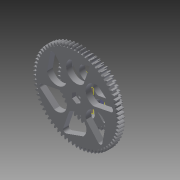
# Autodesk Inventor part: quarterinch-cap
Saved by Autodesk Inventor 2014 (Build 180170000, 170)
## iProperties
Created: 2013-11-06
Part Number: quarterinch-cap
Material: Generic
Document SubType Name: Modeling
Designer: stephen
Density: 1 g/cm^3
Appearance: Default
Author: stephen
Autodesk Inventor part; units mm, degrees
(part 1 of 2)
ref_plane "YZ Plane" through (0, 0, 0) normal (1, 0, 0) x (0, 1, 0)
ref_plane "XZ Plane" through (0, 0, 0) normal (0, 1, 0) x (-1, 0, 0)
ref_plane "XY Plane" through (0, 0, 0) normal (0, 0, 1) x (1, 0, 0)
ref_plane "Work Plane10" through (2.7665, 46.0619, 25.38) normal (0, 0, 1) x (1, 0, 0)
sketch "Sketch15" plane through (2.7665, 46.0619, 25.38) normal (0, 0, 1) x (1, 0, 0)
  line L0 (-0.1767, 42.3028) -> (0.1689, 42.3028)
  arc A0 (0.9579, 39.3583) -> (0.1689, 42.3028) centre (-2.8295, 39.9215) ccw
  line L1 (0.1689, 42.3028) -> (0.9579, 39.3583) construction
  arc A1 (-0.1767, 42.3028) -> (-0.9656, 39.3582) centre (2.8217, 39.9215) ccw
  line L2 (-3.968, 42.1167) -> (-3.6238, 42.1476)
  arc A2 (-2.5741, 39.2858) -> (-3.6238, 42.1476) centre (-6.3966, 39.5071) ccw
  line L3 (-3.6238, 42.1476) -> (-2.5741, 39.2858) construction
  arc A3 (-3.968, 42.1167) -> (-4.4898, 39.1132) centre (-0.7682, 40.0137) ccw
  line L4 (-7.7273, 41.5914) -> (-7.3873, 41.6531)
  arc A4 (-6.0852, 38.8969) -> (-7.3873, 41.6531) centre (-9.9122, 38.7747) ccw
  line L5 (-7.3873, 41.6531) -> (-6.0852, 38.8969) construction
  arc A5 (-7.7273, 41.5914) -> (-7.9778, 38.5532) centre (-4.3519, 39.7837) ccw
  line L6 (-11.4244, 40.7313) -> (-11.0913, 40.8233)
  arc A6 (-9.5474, 38.1948) -> (-11.0913, 40.8233) centre (-13.3481, 37.7301) ccw
  line L7 (-11.0913, 40.8233) -> (-9.5474, 38.1948) construction
  arc A7 (-11.4244, 40.7313) -> (-11.4015, 37.6829) centre (-7.9006, 39.2335) ccw
  line L8 (-15.0295, 39.5433) -> (-14.706, 39.6647)
  arc A8 (-12.9328, 37.1852) -> (-14.706, 39.6647) centre (-16.6764, 36.3817) ccw
  line L9 (-14.706, 39.6647) -> (-12.9328, 37.1852) construction
  arc A9 (-15.0295, 39.5433) -> (-14.7335, 36.5092) centre (-11.3856, 38.3673) ccw
  line L10 (-18.5137, 38.0368) -> (-18.2023, 38.1868)
  arc A10 (-16.2139, 35.8762) -> (-18.2023, 38.1868) centre (-19.8705, 34.7403) ccw
  line L11 (-18.2023, 38.1868) -> (-16.2139, 35.8762) construction
  arc A11 (-18.5137, 38.0368) -> (-17.9468, 35.0415) centre (-14.779, 37.1923) ccw
  line L12 (-21.8487, 36.2242) -> (-21.5521, 36.4014)
  arc A12 (-19.3646, 34.2784) -> (-21.5521, 36.4014) centre (-22.9046, 32.8193) ccw
  line L13 (-21.5521, 36.4014) -> (-19.3646, 34.2784) construction
  arc A13 (-21.8487, 36.2242) -> (-21.0157, 33.2917) centre (-18.0534, 35.7178) ccw
  line L14 (-25.0079, 34.1198) -> (-24.7283, 34.323)
  arc A14 (-22.3593, 32.4046) -> (-24.7283, 34.323) centre (-25.7543, 30.634) ccw
  line L15 (-24.7283, 34.323) -> (-22.3593, 32.4046) construction
  arc A15 (-25.0079, 34.1198) -> (-23.9153, 31.2738) centre (-21.1825, 33.9557) ccw
  line L16 (-27.9657, 31.7408) -> (-27.7055, 31.9681)
  arc A16 (-25.174, 30.2699) -> (-27.7055, 31.9681) centre (-28.3967, 28.2021) ccw
  line L17 (-27.7055, 31.9681) -> (-25.174, 30.2699) construction
  arc A17 (-27.9657, 31.7408) -> (-26.6224, 29.0042) centre (-24.1409, 31.9202) ccw
  line L18 (-30.6983, 29.1062) -> (-30.4595, 29.356)
  arc A18 (-27.7861, 27.8914) -> (-30.4595, 29.356) centre (-30.8104, 25.5431) ccw
  line L19 (-30.4595, 29.356) -> (-27.7861, 27.8914) construction
  arc A19 (-30.6983, 29.1062) -> (-29.1152, 26.501) centre (-26.9051, 29.6277) ccw
  line L20 (-33.1838, 26.2372) -> (-32.9683, 26.5074)
  arc A20 (-30.1744, 25.2884) -> (-32.9683, 26.5074) centre (-32.976, 22.6785) ccw
  line L21 (-32.9683, 26.5074) -> (-30.1744, 25.2884) construction
  arc A21 (-33.1838, 26.2372) -> (-31.3735, 23.7845) centre (-29.4526, 27.0967) ccw
  line L22 (-35.4021, 23.157) -> (-35.2117, 23.4454)
  arc A22 (-32.3197, 22.4818) -> (-35.2117, 23.4454) centre (-34.8761, 19.6312) ccw
  line L23 (-35.2117, 23.4454) -> (-32.3197, 22.4818) construction
  arc A23 (-35.4021, 23.157) -> (-33.3792, 20.8764) centre (-31.7629, 24.3475) ccw
  line L24 (-37.3354, 19.8904) -> (-37.1716, 20.1947)
  arc A24 (-34.2049, 19.4942) -> (-37.1716, 20.1947) centre (-36.4955, 16.4259) ccw
  line L25 (-37.1716, 20.1947) -> (-34.2049, 19.4942) construction
  arc A25 (-37.3354, 19.8904) -> (-35.1162, 17.8003) centre (-33.8176, 21.4023) ccw
  line L26 (-38.968, 16.4636) -> (-38.8322, 16.7814)
  arc A26 (-35.8146, 16.3496) -> (-38.8322, 16.7814) centre (-37.8209, 13.0884) ccw
  line L27 (-38.8322, 16.7814) -> (-35.8146, 16.3496) construction
  arc A27 (-38.968, 16.4636) -> (-36.5704, 14.5808) centre (-35.5999, 18.2847) ccw
  line L28 (-40.2869, 12.9043) -> (-40.1802, 13.2329)
  arc A28 (-37.136, 13.0734) -> (-40.1802, 13.2329) centre (-38.8419, 9.6454) ccw
  line L29 (-40.1802, 13.2329) -> (-37.136, 13.0734) construction
  arc A29 (-40.2869, 12.9043) -> (-37.7302, 11.244) centre (-37.0956, 15.02) ccw
  line L30 (-41.2815, 9.241) -> (-41.2046, 9.5779)
  arc A30 (-38.1584, 9.6919) -> (-41.2046, 9.5779) centre (-39.5502, 6.1248) ccw
  line L31 (-41.2046, 9.5779) -> (-38.1584, 9.6919) construction
  arc A31 (-41.2815, 9.241) -> (-38.5862, 7.8166) centre (-38.2927, 11.6343) ccw
  line L32 (-41.9437, 5.5034) -> (-41.8973, 5.8458)
  arc A32 (-38.8736, 6.2324) -> (-41.8973, 5.8458) centre (-39.94, 2.5549) ccw
  line L33 (-41.8973, 5.8458) -> (-38.8736, 6.2324) construction
  arc A33 (-41.9437, 5.5034) -> (-39.1316, 4.3263) centre (-39.1814, 8.1549) ccw
  line L34 (-42.2681, 1.7214) -> (-42.2526, 2.0666)
  arc A34 (-39.2757, 2.7227) -> (-42.2526, 2.0666) centre (-40.0082, -1.0355) ccw
  line L35 (-42.2526, 2.0666) -> (-39.2757, 2.7227) construction
  arc A35 (-42.2681, 1.7214) -> (-39.3618, 0.8012) centre (-39.7547, 4.6099) ccw
  line L36 (-42.2523, -2.0744) -> (-42.2678, -1.7292)
  arc A36 (-39.3617, -0.8089) -> (-42.2678, -1.7292) centre (-39.7543, -4.6177) ccw
  line L37 (-42.2678, -1.7292) -> (-39.3617, -0.8089) construction
  arc A37 (-42.2523, -2.0744) -> (-39.2752, -2.7304) centre (-40.0079, 1.0278) ccw
  line L38 (-41.8962, -5.8535) -> (-41.9426, -5.5111)
  arc A38 (-39.1307, -4.334) -> (-41.9426, -5.5111) centre (-39.1804, -8.1626) ccw
  line L39 (-41.9426, -5.5111) -> (-39.1307, -4.334) construction
  arc A39 (-41.8962, -5.8535) -> (-38.8723, -6.24) centre (-39.9389, -2.5626) ccw
  line L40 (-41.2029, -9.5855) -> (-41.2798, -9.2486)
  arc A40 (-38.5847, -7.8242) -> (-41.2798, -9.2486) centre (-38.2909, -11.6419) ccw
  line L41 (-41.2798, -9.2486) -> (-38.5847, -7.8242) construction
  arc A41 (-41.2029, -9.5855) -> (-38.1565, -9.6994) centre (-39.5484, -6.1324) ccw
  line L42 (-40.1777, -13.2403) -> (-40.2845, -12.9117)
  arc A42 (-37.728, -11.2514) -> (-40.2845, -12.9117) centre (-37.0932, -15.0274) ccw
  line L43 (-40.2845, -12.9117) -> (-37.728, -11.2514) construction
  arc A43 (-40.1777, -13.2403) -> (-37.1334, -13.0807) centre (-38.8395, -9.6528) ccw
  line L44 (-38.8292, -16.7885) -> (-38.965, -16.4708)
  arc A44 (-36.5676, -14.588) -> (-38.965, -16.4708) centre (-35.5968, -18.2919) ccw
  line L45 (-38.965, -16.4708) -> (-36.5676, -14.588) construction
  arc A45 (-38.8292, -16.7885) -> (-35.8114, -16.3566) centre (-37.8179, -13.0955) ccw
  line L46 (-37.1679, -20.2015) -> (-37.3317, -19.8972)
  arc A46 (-35.1127, -17.8072) -> (-37.3317, -19.8972) centre (-33.8139, -21.4091) ccw
  line L47 (-37.3317, -19.8972) -> (-35.1127, -17.8072) construction
  arc A47 (-37.1679, -20.2015) -> (-34.201, -19.5009) centre (-36.4918, -16.4328) ccw
  line L48 (-35.2074, -23.4519) -> (-35.3978, -23.1635)
  arc A48 (-33.3751, -20.883) -> (-35.3978, -23.1635) centre (-31.7586, -24.354) ccw
  line L49 (-35.3978, -23.1635) -> (-33.3751, -20.883) construction
  arc A49 (-35.2074, -23.4519) -> (-32.3153, -22.4882) centre (-34.8718, -19.6377) ccw
  line L50 (-32.9635, -26.5135) -> (-33.179, -26.2433)
  arc A50 (-31.3688, -23.7906) -> (-33.179, -26.2433) centre (-29.4477, -27.1028) ccw
  line L51 (-33.179, -26.2433) -> (-31.3688, -23.7906) construction
  arc A51 (-32.9635, -26.5135) -> (-30.1694, -25.2944) centre (-32.9711, -22.6845) ccw
  line L52 (-30.4541, -29.3616) -> (-30.693, -29.1118)
  arc A52 (-29.1099, -26.5067) -> (-30.693, -29.1118) centre (-26.8997, -29.6333) ccw
  line L53 (-30.693, -29.1118) -> (-29.1099, -26.5067) construction
  arc A53 (-30.4541, -29.3616) -> (-27.7806, -27.8969) centre (-30.805, -25.5487) ccw
  line L54 (-27.6996, -31.9733) -> (-27.9598, -31.7459)
  arc A54 (-26.6167, -29.0094) -> (-27.9598, -31.7459) centre (-24.1351, -31.9253) ccw
  line L55 (-27.9598, -31.7459) -> (-26.6167, -29.0094) construction
  arc A55 (-27.6996, -31.9733) -> (-25.1681, -30.2748) centre (-28.3908, -28.2072) ccw
  line L56 (-24.722, -34.3275) -> (-25.0016, -34.1244)
  arc A56 (-23.9092, -31.2786) -> (-25.0016, -34.1244) centre (-21.1762, -33.9603) ccw
  line L57 (-25.0016, -34.1244) -> (-23.9092, -31.2786) construction
  arc A57 (-24.722, -34.3275) -> (-22.3529, -32.409) centre (-25.748, -30.6386) ccw
  line L58 (-21.5454, -36.4054) -> (-21.8421, -36.2282)
  arc A58 (-21.0091, -33.2958) -> (-21.8421, -36.2282) centre (-18.0467, -35.7218) ccw
  line L59 (-21.8421, -36.2282) -> (-21.0091, -33.2958) construction
  arc A59 (-21.5454, -36.4054) -> (-19.3578, -34.2822) centre (-22.898, -32.8233) ccw
  line L60 (-18.1953, -38.1902) -> (-18.5067, -38.0402)
  arc A60 (-17.9399, -35.045) -> (-18.5067, -38.0402) centre (-14.772, -37.1956) ccw
  line L61 (-18.5067, -38.0402) -> (-17.9399, -35.045) construction
  arc A61 (-18.1953, -38.1902) -> (-16.2069, -35.8794) centre (-19.8635, -34.7437) ccw
  line L62 (-14.6987, -39.6674) -> (-15.0223, -39.546)
  arc A62 (-14.7263, -36.5121) -> (-15.0223, -39.546) centre (-11.3784, -38.3701) ccw
  line L63 (-15.0223, -39.546) -> (-14.7263, -36.5121) construction
  arc A63 (-14.6987, -39.6674) -> (-12.9254, -37.1878) centre (-16.6692, -36.3844) ccw
  line L64 (-11.0838, -40.8253) -> (-11.4169, -40.7334)
  arc A64 (-11.3941, -37.6852) -> (-11.4169, -40.7334) centre (-7.8931, -39.2355) ccw
  line L65 (-11.4169, -40.7334) -> (-11.3941, -37.6852) construction
  arc A65 (-11.0838, -40.8253) -> (-9.5399, -38.1967) centre (-13.3406, -37.7321) ccw
  line L66 (-7.3796, -41.6545) -> (-7.7196, -41.5928)
  arc A66 (-7.9702, -38.5548) -> (-7.7196, -41.5928) centre (-4.3443, -39.7851) ccw
  line L67 (-7.7196, -41.5928) -> (-7.9702, -38.5548) construction
  arc A67 (-7.3796, -41.6545) -> (-6.0776, -38.8981) centre (-9.9046, -38.7761) ccw
  line L68 (-3.616, -42.1483) -> (-3.9602, -42.1174)
  arc A68 (-4.4821, -39.114) -> (-3.9602, -42.1174) centre (-0.7605, -40.0144) ccw
  line L69 (-3.9602, -42.1174) -> (-4.4821, -39.114) construction
  arc A69 (-3.616, -42.1483) -> (-2.5663, -39.2863) centre (-6.3889, -39.5078) ccw
  line L70 (0.1767, -42.3028) -> (-0.1689, -42.3028)
  arc A70 (-0.9579, -39.3583) -> (-0.1689, -42.3028) centre (2.8295, -39.9215) ccw
  line L71 (-0.1689, -42.3028) -> (-0.9579, -39.3583) construction
  arc A71 (0.1767, -42.3028) -> (0.9656, -39.3582) centre (-2.8217, -39.9215) ccw
  line L72 (3.968, -42.1167) -> (3.6238, -42.1476)
  arc A72 (2.5741, -39.2858) -> (3.6238, -42.1476) centre (6.3966, -39.5071) ccw
  line L73 (3.6238, -42.1476) -> (2.5741, -39.2858) construction
  arc A73 (3.968, -42.1167) -> (4.4898, -39.1132) centre (0.7682, -40.0137) ccw
  line L74 (7.7273, -41.5914) -> (7.3873, -41.6531)
  arc A74 (6.0852, -38.8969) -> (7.3873, -41.6531) centre (9.9122, -38.7747) ccw
  line L75 (7.3873, -41.6531) -> (6.0852, -38.8969) construction
  arc A75 (7.7273, -41.5914) -> (7.9778, -38.5532) centre (4.3519, -39.7837) ccw
  line L76 (11.4244, -40.7313) -> (11.0913, -40.8233)
  arc A76 (9.5474, -38.1948) -> (11.0913, -40.8233) centre (13.3481, -37.7301) ccw
  line L77 (11.0913, -40.8233) -> (9.5474, -38.1948) construction
  arc A77 (11.4244, -40.7313) -> (11.4015, -37.6829) centre (7.9006, -39.2335) ccw
  line L78 (15.0295, -39.5433) -> (14.706, -39.6647)
  arc A78 (12.9328, -37.1852) -> (14.706, -39.6647) centre (16.6764, -36.3817) ccw
  line L79 (14.706, -39.6647) -> (12.9328, -37.1852) construction
  arc A79 (15.0295, -39.5433) -> (14.7335, -36.5092) centre (11.3856, -38.3673) ccw
  line L80 (18.5137, -38.0368) -> (18.2023, -38.1868)
  arc A80 (16.2139, -35.8762) -> (18.2023, -38.1868) centre (19.8705, -34.7403) ccw
  line L81 (18.2023, -38.1868) -> (16.2139, -35.8762) construction
  arc A81 (18.5137, -38.0368) -> (17.9468, -35.0415) centre (14.779, -37.1923) ccw
  line L82 (21.8487, -36.2242) -> (21.5521, -36.4014)
  arc A82 (19.3646, -34.2784) -> (21.5521, -36.4014) centre (22.9046, -32.8193) ccw
  line L83 (21.5521, -36.4014) -> (19.3646, -34.2784) construction
  arc A83 (21.8487, -36.2242) -> (21.0157, -33.2917) centre (18.0534, -35.7178) ccw
  line L84 (25.0079, -34.1198) -> (24.7283, -34.323)
  arc A84 (22.3593, -32.4046) -> (24.7283, -34.323) centre (25.7543, -30.634) ccw
  line L85 (24.7283, -34.323) -> (22.3593, -32.4046) construction
  arc A85 (25.0079, -34.1198) -> (23.9153, -31.2738) centre (21.1825, -33.9557) ccw
  line L86 (27.9657, -31.7408) -> (27.7055, -31.9681)
  arc A86 (25.174, -30.2699) -> (27.7055, -31.9681) centre (28.3967, -28.2021) ccw
  line L87 (27.7055, -31.9681) -> (25.174, -30.2699) construction
  arc A87 (27.9657, -31.7408) -> (26.6224, -29.0042) centre (24.1409, -31.9202) ccw
  line L88 (30.6983, -29.1062) -> (30.4595, -29.356)
  arc A88 (27.7861, -27.8914) -> (30.4595, -29.356) centre (30.8104, -25.5431) ccw
  line L89 (30.4595, -29.356) -> (27.7861, -27.8914) construction
  arc A89 (30.6983, -29.1062) -> (29.1152, -26.501) centre (26.9051, -29.6277) ccw
  line L90 (33.1838, -26.2372) -> (32.9683, -26.5074)
  arc A90 (30.1744, -25.2884) -> (32.9683, -26.5074) centre (32.976, -22.6785) ccw
  line L91 (32.9683, -26.5074) -> (30.1744, -25.2884) construction
  arc A91 (33.1838, -26.2372) -> (31.3735, -23.7845) centre (29.4526, -27.0967) ccw
  line L92 (35.4021, -23.157) -> (35.2117, -23.4454)
  arc A92 (32.3197, -22.4818) -> (35.2117, -23.4454) centre (34.8761, -19.6312) ccw
  line L93 (35.2117, -23.4454) -> (32.3197, -22.4818) construction
  arc A93 (35.4021, -23.157) -> (33.3792, -20.8764) centre (31.7629, -24.3475) ccw
  line L94 (37.3354, -19.8904) -> (37.1716, -20.1947)
  arc A94 (34.2049, -19.4942) -> (37.1716, -20.1947) centre (36.4955, -16.4259) ccw
  line L95 (37.1716, -20.1947) -> (34.2049, -19.4942) construction
  arc A95 (37.3354, -19.8904) -> (35.1162, -17.8003) centre (33.8176, -21.4023) ccw
  line L96 (38.968, -16.4636) -> (38.8322, -16.7814)
  arc A96 (35.8146, -16.3496) -> (38.8322, -16.7814) centre (37.8209, -13.0884) ccw
  line L97 (38.8322, -16.7814) -> (35.8146, -16.3496) construction
  arc A97 (38.968, -16.4636) -> (36.5704, -14.5808) centre (35.5999, -18.2847) ccw
  line L98 (40.2869, -12.9043) -> (40.1802, -13.2329)
  arc A98 (37.136, -13.0734) -> (40.1802, -13.2329) centre (38.8419, -9.6454) ccw
  line L99 (40.1802, -13.2329) -> (37.136, -13.0734) construction
  arc A99 (40.2869, -12.9043) -> (37.7302, -11.244) centre (37.0956, -15.02) ccw
  line L100 (41.2815, -9.241) -> (41.2046, -9.5779)
  arc A100 (38.1584, -9.6919) -> (41.2046, -9.5779) centre (39.5502, -6.1248) ccw
  line L101 (41.2046, -9.5779) -> (38.1584, -9.6919) construction
  arc A101 (41.2815, -9.241) -> (38.5862, -7.8166) centre (38.2927, -11.6343) ccw
  line L102 (41.9437, -5.5034) -> (41.8973, -5.8458)
  arc A102 (38.8736, -6.2324) -> (41.8973, -5.8458) centre (39.94, -2.5549) ccw
  line L103 (41.8973, -5.8458) -> (38.8736, -6.2324) construction
  arc A103 (41.9437, -5.5034) -> (39.1316, -4.3263) centre (39.1814, -8.1549) ccw
  line L104 (42.2681, -1.7214) -> (42.2526, -2.0666)
  arc A104 (39.2757, -2.7227) -> (42.2526, -2.0666) centre (40.0082, 1.0355) ccw
  line L105 (42.2526, -2.0666) -> (39.2757, -2.7227) construction
  arc A105 (42.2681, -1.7214) -> (39.3618, -0.8012) centre (39.7547, -4.6099) ccw
  line L106 (42.2523, 2.0744) -> (42.2678, 1.7292)
  arc A106 (39.3617, 0.8089) -> (42.2678, 1.7292) centre (39.7543, 4.6177) ccw
  line L107 (42.2678, 1.7292) -> (39.3617, 0.8089) construction
  arc A107 (42.2523, 2.0744) -> (39.2752, 2.7304) centre (40.0079, -1.0278) ccw
  line L108 (41.8962, 5.8535) -> (41.9426, 5.5111)
  arc A108 (39.1307, 4.334) -> (41.9426, 5.5111) centre (39.1804, 8.1626) ccw
  line L109 (41.9426, 5.5111) -> (39.1307, 4.334) construction
  arc A109 (41.8962, 5.8535) -> (38.8723, 6.24) centre (39.9389, 2.5626) ccw
  line L110 (41.2029, 9.5855) -> (41.2798, 9.2486)
  arc A110 (38.5847, 7.8242) -> (41.2798, 9.2486) centre (38.2909, 11.6419) ccw
  line L111 (41.2798, 9.2486) -> (38.5847, 7.8242) construction
  arc A111 (41.2029, 9.5855) -> (38.1565, 9.6994) centre (39.5484, 6.1324) ccw
  line L112 (40.1777, 13.2403) -> (40.2845, 12.9117)
  arc A112 (37.728, 11.2514) -> (40.2845, 12.9117) centre (37.0932, 15.0274) ccw
  line L113 (40.2845, 12.9117) -> (37.728, 11.2514) construction
  arc A113 (40.1777, 13.2403) -> (37.1334, 13.0807) centre (38.8395, 9.6528) ccw
  line L114 (38.8292, 16.7885) -> (38.965, 16.4708)
  arc A114 (36.5676, 14.588) -> (38.965, 16.4708) centre (35.5968, 18.2919) ccw
  line L115 (38.965, 16.4708) -> (36.5676, 14.588) construction
  arc A115 (38.8292, 16.7885) -> (35.8114, 16.3566) centre (37.8179, 13.0955) ccw
  line L116 (37.1679, 20.2015) -> (37.3317, 19.8972)
  arc A116 (35.1127, 17.8072) -> (37.3317, 19.8972) centre (33.8139, 21.4091) ccw
  line L117 (37.3317, 19.8972) -> (35.1127, 17.8072) construction
  arc A117 (37.1679, 20.2015) -> (34.201, 19.5009) centre (36.4918, 16.4328) ccw
  line L118 (35.2074, 23.4519) -> (35.3978, 23.1635)
  arc A118 (33.3751, 20.883) -> (35.3978, 23.1635) centre (31.7586, 24.354) ccw
  line L119 (35.3978, 23.1635) -> (33.3751, 20.883) construction
  arc A119 (35.2074, 23.4519) -> (32.3153, 22.4882) centre (34.8718, 19.6377) ccw
  line L120 (32.9635, 26.5135) -> (33.179, 26.2433)
  arc A120 (31.3688, 23.7906) -> (33.179, 26.2433) centre (29.4477, 27.1028) ccw
  line L121 (33.179, 26.2433) -> (31.3688, 23.7906) construction
  arc A121 (32.9635, 26.5135) -> (30.1694, 25.2944) centre (32.9711, 22.6845) ccw
  line L122 (30.4541, 29.3616) -> (30.693, 29.1118)
  arc A122 (29.1099, 26.5067) -> (30.693, 29.1118) centre (26.8997, 29.6333) ccw
  line L123 (30.693, 29.1118) -> (29.1099, 26.5067) construction
  arc A123 (30.4541, 29.3616) -> (27.7806, 27.8969) centre (30.805, 25.5487) ccw
  line L124 (27.6996, 31.9733) -> (27.9598, 31.7459)
  arc A124 (26.6167, 29.0094) -> (27.9598, 31.7459) centre (24.1351, 31.9253) ccw
  line L125 (27.9598, 31.7459) -> (26.6167, 29.0094) construction
  arc A125 (27.6996, 31.9733) -> (25.1681, 30.2748) centre (28.3908, 28.2072) ccw
  line L126 (24.722, 34.3275) -> (25.0016, 34.1244)
  arc A126 (23.9092, 31.2786) -> (25.0016, 34.1244) centre (21.1762, 33.9603) ccw
  line L127 (25.0016, 34.1244) -> (23.9092, 31.2786) construction
  arc A127 (24.722, 34.3275) -> (22.3529, 32.409) centre (25.748, 30.6386) ccw
  line L128 (21.5454, 36.4054) -> (21.8421, 36.2282)
  arc A128 (21.0091, 33.2958) -> (21.8421, 36.2282) centre (18.0467, 35.7218) ccw
  line L129 (21.8421, 36.2282) -> (21.0091, 33.2958) construction
  arc A129 (21.5454, 36.4054) -> (19.3578, 34.2822) centre (22.898, 32.8233) ccw
  line L130 (18.1953, 38.1902) -> (18.5067, 38.0402)
  arc A130 (17.9399, 35.045) -> (18.5067, 38.0402) centre (14.772, 37.1956) ccw
  line L131 (18.5067, 38.0402) -> (17.9399, 35.045) construction
  arc A131 (18.1953, 38.1902) -> (16.2069, 35.8794) centre (19.8635, 34.7437) ccw
  line L132 (14.6987, 39.6674) -> (15.0223, 39.546)
  arc A132 (14.7263, 36.5121) -> (15.0223, 39.546) centre (11.3784, 38.3701) ccw
  line L133 (15.0223, 39.546) -> (14.7263, 36.5121) construction
  arc A133 (14.6987, 39.6674) -> (12.9254, 37.1878) centre (16.6692, 36.3844) ccw
  line L134 (11.0838, 40.8253) -> (11.4169, 40.7334)
  arc A134 (11.3941, 37.6852) -> (11.4169, 40.7334) centre (7.8931, 39.2355) ccw
  line L135 (11.4169, 40.7334) -> (11.3941, 37.6852) construction
  arc A135 (11.0838, 40.8253) -> (9.5399, 38.1967) centre (13.3406, 37.7321) ccw
  line L136 (7.3796, 41.6545) -> (7.7196, 41.5928)
  arc A136 (7.9702, 38.5548) -> (7.7196, 41.5928) centre (4.3443, 39.7851) ccw
  line L137 (7.7196, 41.5928) -> (7.9702, 38.5548) construction
  arc A137 (7.3796, 41.6545) -> (6.0776, 38.8981) centre (9.9046, 38.7761) ccw
  line L138 (3.616, 42.1483) -> (3.9602, 42.1174)
  arc A138 (4.4821, 39.114) -> (3.9602, 42.1174) centre (0.7605, 40.0144) ccw
  line L139 (3.9602, 42.1174) -> (4.4821, 39.114) construction
  arc A139 (3.616, 42.1483) -> (2.5663, 39.2863) centre (6.3889, 39.5078) ccw
  line L140 (73.0043, -23.5061) -> (73.0043, 76.8994)
  line L141 (73.0043, -23.5061) -> (-27.4013, -23.5061) construction
  line L142 (12.7685, 31.9695) -> (7.0232, 15.0428)
  line L143 (-7.0232, 29.0892) -> (9.6761, 35.0189)
  arc A140 (-7.0232, 29.0892) -> (7.0232, 15.0428) centre (0, 22.066) ccw
  arc A141 (12.7685, 31.9695) -> (9.6761, 35.0189) centre (10.4835, 32.745) ccw
  line L144 (34.1169, 4.9001) -> (16.5854, 1.4124)
  arc A142 (21.7267, 20.6) -> (16.5854, 1.4124) centre (19.1561, 11.0062) ccw
  line L145 (21.7267, 20.6) -> (35.2117, 9.103)
  arc A143 (34.1169, 4.9001) -> (35.2117, 9.103) centre (33.6461, 7.2667) ccw
  line L146 (21.3176, -27.0693) -> (9.5313, -13.6305)
  arc A144 (28.719, -8.4891) -> (9.5313, -13.6305) centre (19.1252, -11.0598) ccw
  line L147 (28.719, -8.4891) -> (25.5047, -25.916)
  arc A145 (21.3176, -27.0693) -> (25.5047, -25.916) centre (23.1317, -25.4783) ccw
  line L148 (-12.7685, -31.9695) -> (-7.0232, -15.0428)
  arc A146 (7.0232, -29.0892) -> (-7.0232, -15.0428) centre (0, -22.066) ccw
  line L149 (7.0232, -29.0892) -> (-9.6761, -35.0189)
  arc A147 (-12.7685, -31.9695) -> (-9.6761, -35.0189) centre (-10.4835, -32.745) ccw
  line L150 (-34.0551, -4.9002) -> (-16.5236, -1.4124)
  arc A148 (-21.6649, -20.6001) -> (-16.5236, -1.4124) centre (-19.0942, -11.0062) ccw
  line L151 (-21.6649, -20.6001) -> (-35.1498, -9.103)
  arc A149 (-34.0551, -4.9002) -> (-35.1498, -9.103) centre (-33.5843, -7.2668) ccw
  line L152 (-21.2557, 27.0693) -> (-9.4695, 13.6304)
  arc A150 (-28.6572, 8.489) -> (-9.4695, 13.6304) centre (-19.0633, 11.0597) ccw
  line L153 (-28.6572, 8.489) -> (-25.4429, 25.9159)
  arc A151 (-21.2557, 27.0693) -> (-25.4429, 25.9159) centre (-23.0699, 25.4782) ccw
  line L154 (11.0838, 0) -> (38.8367, 0) construction
  line L155 (0, 0) -> (0, -16.4636)
  line L156 (0, 0) -> (9.5313, 0)
  line L157 (11.0838, 0) -> (9.4861, 0)
  line L158 (2.4848, 0) -> (0, 0)
  line L159 (0, 0) -> (0, -5.6488)
  line L160 (0, -11.1197) -> (0, -12.1337)
  arc A152 (-32.3153, -22.4882) -> (-31.3688, -23.7906) centre (0, 0) ccw
  arc A153 (-34.201, -19.5009) -> (-33.3751, -20.883) centre (0, 0) ccw
  arc A154 (-35.8114, -16.3566) -> (-35.1127, -17.8072) centre (0, 0) ccw
  arc A155 (-37.1334, -13.0807) -> (-36.5676, -14.588) centre (0, 0) ccw
  arc A156 (-38.8723, -6.24) -> (-38.5847, -7.8242) centre (0, 0) ccw
  arc A157 (-38.1565, -9.6994) -> (-37.728, -11.2514) centre (0, 0) ccw
  arc A158 (-39.2752, -2.7304) -> (-39.1307, -4.334) centre (0, 0) ccw
  arc A159 (-39.3618, 0.8012) -> (-39.3617, -0.8089) centre (0, 0) ccw
  arc A160 (-39.1316, 4.3263) -> (-39.2757, 2.7227) centre (0, 0) ccw
  arc A161 (-38.5862, 7.8166) -> (-38.8736, 6.2324) centre (0, 0) ccw
  arc A162 (-37.7302, 11.244) -> (-38.1584, 9.6919) centre (0, 0) ccw
  arc A163 (-36.5704, 14.5808) -> (-37.136, 13.0734) centre (0, 0) ccw
  arc A164 (-35.1162, 17.8003) -> (-35.8146, 16.3496) centre (0, 0) ccw
  arc A165 (-30.1694, -25.2944) -> (-29.1099, -26.5067) centre (0, 0) ccw
  arc A166 (-27.7806, -27.8969) -> (-26.6167, -29.0094) centre (0, 0) ccw
  arc A167 (-25.1681, -30.2748) -> (-23.9092, -31.2786) centre (0, 0) ccw
  arc A168 (-22.3529, -32.409) -> (-21.0091, -33.2958) centre (0, 0) ccw
  arc A169 (-19.3578, -34.2822) -> (-17.9399, -35.045) centre (0, 0) ccw
  arc A170 (-16.2069, -35.8794) -> (-14.7263, -36.5121) centre (0, 0) ccw
  arc A171 (-12.9254, -37.1878) -> (-11.3941, -37.6852) centre (0, 0) ccw
  arc A172 (-9.5399, -38.1967) -> (-7.9702, -38.5548) centre (0, 0) ccw
  arc A173 (-6.0776, -38.8981) -> (-4.4821, -39.114) centre (0, 0) ccw
  arc A174 (-2.5663, -39.2863) -> (-0.9579, -39.3583) centre (0, 0) ccw
  arc A175 (-33.3792, 20.8764) -> (-34.2049, 19.4942) centre (0, 0) ccw
  arc A176 (-31.3735, 23.7845) -> (-32.3197, 22.4818) centre (0, 0) ccw
  arc A177 (-29.1152, 26.501) -> (-30.1744, 25.2884) centre (0, 0) ccw
  arc A178 (-26.6224, 29.0042) -> (-27.7861, 27.8914) centre (0, 0) ccw
  arc A179 (-23.9153, 31.2738) -> (-25.174, 30.2699) centre (0, 0) ccw
  arc A180 (-21.0157, 33.2917) -> (-22.3593, 32.4046) centre (0, 0) ccw
  arc A181 (-17.9468, 35.0415) -> (-19.3646, 34.2784) centre (0, 0) ccw
  arc A182 (-14.7335, 36.5092) -> (-16.2139, 35.8762) centre (0, 0) ccw
  arc A183 (-11.4015, 37.6829) -> (-12.9328, 37.1852) centre (0, 0) ccw
  arc A184 (-7.9778, 38.5532) -> (-9.5474, 38.1948) centre (0, 0) ccw
  arc A185 (-4.4898, 39.1132) -> (-6.0852, 38.8969) centre (0, 0) ccw
  arc A186 (-0.9656, 39.3582) -> (-2.5741, 39.2858) centre (0, 0) ccw
  arc A187 (2.5663, 39.2863) -> (0.9579, 39.3583) centre (0, 0) ccw
  arc A188 (6.0776, 38.8981) -> (4.4821, 39.114) centre (0, 0) ccw
  arc A189 (9.5399, 38.1967) -> (7.9702, 38.5548) centre (0, 0) ccw
  arc A190 (12.9254, 37.1878) -> (11.3941, 37.6852) centre (0, 0) ccw
  arc A191 (16.2069, 35.8794) -> (14.7263, 36.5121) centre (0, 0) ccw
  arc A192 (19.3578, 34.2822) -> (17.9399, 35.045) centre (0, 0) ccw
  arc A193 (22.3529, 32.409) -> (21.0091, 33.2958) centre (0, 0) ccw
  arc A194 (25.1681, 30.2748) -> (23.9092, 31.2786) centre (0, 0) ccw
  arc A195 (27.7806, 27.8969) -> (26.6167, 29.0094) centre (0, 0) ccw
  arc A196 (30.1694, 25.2944) -> (29.1099, 26.5067) centre (0, 0) ccw
  arc A197 (32.3153, 22.4882) -> (31.3688, 23.7906) centre (0, 0) ccw
  arc A198 (34.201, 19.5009) -> (33.3751, 20.883) centre (0, 0) ccw
  arc A199 (35.8114, 16.3566) -> (35.1127, 17.8072) centre (0, 0) ccw
  arc A200 (37.1334, 13.0807) -> (36.5676, 14.588) centre (0, 0) ccw
  arc A201 (38.1565, 9.6994) -> (37.728, 11.2514) centre (0, 0) ccw
  arc A202 (38.8723, 6.24) -> (38.5847, 7.8242) centre (0, 0) ccw
  arc A203 (39.2752, 2.7304) -> (39.1307, 4.334) centre (0, 0) ccw
  arc A204 (39.3618, -0.8012) -> (39.3617, 0.8089) centre (0, 0) ccw
  arc A205 (39.1316, -4.3263) -> (39.2757, -2.7227) centre (0, 0) ccw
  arc A206 (38.5862, -7.8166) -> (38.8736, -6.2324) centre (0, 0) ccw
  arc A207 (37.7302, -11.244) -> (38.1584, -9.6919) centre (0, 0) ccw
  arc A208 (36.5704, -14.5808) -> (37.136, -13.0734) centre (0, 0) ccw
  arc A209 (35.1162, -17.8003) -> (35.8146, -16.3496) centre (0, 0) ccw
  arc A210 (33.3792, -20.8764) -> (34.2049, -19.4942) centre (0, 0) ccw
  arc A211 (31.3735, -23.7845) -> (32.3197, -22.4818) centre (0, 0) ccw
  arc A212 (29.1152, -26.501) -> (30.1744, -25.2884) centre (0, 0) ccw
  arc A213 (26.6224, -29.0042) -> (27.7861, -27.8914) centre (0, 0) ccw
  arc A214 (23.9153, -31.2738) -> (25.174, -30.2699) centre (0, 0) ccw
  arc A215 (21.0157, -33.2917) -> (22.3593, -32.4046) centre (0, 0) ccw
  arc A216 (17.9468, -35.0415) -> (19.3646, -34.2784) centre (0, 0) ccw
  arc A217 (14.7335, -36.5092) -> (16.2139, -35.8762) centre (0, 0) ccw
  arc A218 (11.4015, -37.6829) -> (12.9328, -37.1852) centre (0, 0) ccw
  arc A219 (7.9778, -38.5532) -> (9.5474, -38.1948) centre (0, 0) ccw
  arc A220 (0.9656, -39.3582) -> (2.5741, -39.2858) centre (0, 0) ccw
  arc A221 (4.4898, -39.1132) -> (6.0852, -38.8969) centre (0, 0) ccw
  dimension "d70" = 360
  dimension "d105" = 90
  constraints: 322 end point, 305 point on circle, 152 centre point, 4 perpendicular, 4 point on line, 3 horizontal, 2 collinear, 913 other
  measures "d105" angle of L141 L140
extrude "Extrusion18" add sketch "Sketch15" along normal blind 5.588
ref_plane "Work Plane8" through (2.7665, 46.0619, 14.665) normal (0, 0, -1) x (-1, 0, 0)
sketch "Sketch20" plane through (2.7665, 46.0619, 14.665) normal (0, 0, -1) x (-1, 0, 0)
  circle A0 centre (0, 0) radius 7.5 projected
  arc A1 (29.418, 0.0559) -> (26.3016, 0.9693) centre (27.1475, -1.9179) ccw projected
  arc A2 (26.3016, 0.9693) -> (26.2316, 2.1488) centre (0, 0) ccw projected
  arc A3 (26.2316, 2.1488) -> (29.2493, 3.5326) centre (26.586, 5.3583) ccw projected
  line L0 (29.2493, 3.5326) -> (29.1481, 3.9764) projected
  arc A4 (29.1481, 3.9764) -> (25.9377, 4.4663) centre (27.1609, 1.7177) ccw projected
  arc A5 (25.9377, 4.4663) -> (25.7111, 5.626) centre (0, 0) ccw projected
  arc A6 (25.7111, 5.626) -> (28.5175, 7.3996) centre (25.6346, 8.854) ccw projected
  line L1 (28.5175, 7.3996) -> (28.358, 7.826) projected
  arc A7 (28.358, 7.826) -> (25.111, 7.8836) centre (26.6896, 5.3225) ccw projected
  arc A8 (25.111, 7.8836) -> (24.7318, 9.0028) centre (0, 0) ccw projected
  arc A9 (24.7318, 9.0028) -> (27.2767, 11.1346) centre (24.2257, 12.1918) ccw projected
  line L2 (27.2767, 11.1346) -> (27.0619, 11.5359) projected
  arc A10 (27.0619, 11.5359) -> (23.8361, 11.1602) centre (25.742, 8.8324) ccw projected
  arc A11 (23.8361, 11.1602) -> (23.3112, 12.2189) centre (0, 0) ccw projected
  arc A12 (23.3112, 12.2189) -> (25.5493, 14.6709) centre (22.3846, 15.312) ccw projected
  line L3 (25.5493, 14.6709) -> (25.2828, 15.04) projected
  arc A13 (25.2828, 15.04) -> (22.136, 14.2377) centre (24.3351, 12.1847) ccw projected
  arc A14 (22.136, 14.2377) -> (21.4746, 15.2169) centre (0, 0) ccw projected
  arc A15 (21.4746, 15.2169) -> (23.3659, 17.9454) centre (20.144, 18.159) ccw projected
  line L4 (23.3659, 17.9454) -> (23.0526, 18.2757) projected
  arc A16 (23.0526, 18.2757) -> (20.0407, 17.0611) centre (22.4939, 15.3195) ccw projected
  arc A17 (20.0407, 17.0611) -> (19.2548, 17.9434) centre (0, 0) ccw projected
  arc A18 (19.2548, 17.9434) -> (20.7655, 20.8996) centre (17.5439, 20.6819) ccw projected
  line L5 (20.7655, 20.8996) -> (20.411, 21.1852) projected
  arc A19 (20.411, 21.1852) -> (17.5879, 19.58) centre (20.2513, 18.181) ccw projected
  arc A20 (17.5879, 19.58) -> (16.6913, 20.3497) centre (0, 0) ccw projected
  arc A21 (16.6913, 20.3497) -> (17.7946, 23.4809) centre (14.6307, 22.8357) ccw projected
  line L6 (17.7946, 23.4809) -> (17.4052, 23.7167) projected
  arc A22 (17.4052, 23.7167) -> (14.8212, 21.7496) centre (17.6473, 20.718) ccw projected
  arc A23 (14.8212, 21.7496) -> (13.8301, 22.3929) centre (0, 0) ccw projected
  arc A24 (13.8301, 22.3929) -> (14.5061, 25.6432) centre (11.4565, 24.582) ccw projected
  line L7 (14.5061, 25.6432) -> (14.0887, 25.825) projected
  arc A25 (14.0887, 25.825) -> (11.79, 23.531) centre (14.7284, 22.8853) ccw projected
  arc A26 (11.79, 23.531) -> (10.722, 24.0365) centre (0, 0) ccw projected
  arc A27 (10.722, 24.0365) -> (10.9587, 27.3479) centre (8.0778, 25.8897) ccw projected
  line L8 (10.9587, 27.3479) -> (10.5209, 27.4724) projected
  arc A28 (10.5209, 27.4724) -> (8.5485, 24.8925) centre (11.5467, 24.6442) ccw projected
  arc A29 (8.5485, 24.8925) -> (7.4226, 25.2511) centre (0, 0) ccw projected
  arc A30 (7.4226, 25.2511) -> (7.2159, 28.5645) centre (4.555, 26.7354) ccw projected
  line L9 (7.2159, 28.5645) -> (6.7653, 28.6296) projected
  arc A31 (6.7653, 28.6296) -> (5.1544, 25.8098) centre (8.1589, 25.9633) ccw projected
  arc A32 (5.1544, 25.8098) -> (3.9907, 26.0151) centre (0, 0) ccw projected
  arc A33 (3.9907, 26.0151) -> (3.3442, 29.2714) centre (0.9508, 27.1039) ccw projected
  line L10 (3.3442, 29.2714) -> (2.889, 29.2759) projected
  arc A34 (2.889, 29.2759) -> (1.6683, 26.2665) centre (4.6256, 26.8191) ccw projected
  arc A35 (1.6683, 26.2665) -> (0.4876, 26.3149) centre (0, 0) ccw projected
  arc A36 (0.4876, 26.3149) -> (-0.5872, 29.456) centre (-2.6702, 26.9888) ccw projected
  line L11 (-0.5872, 29.456) -> (-1.0389, 29.3997) projected
  arc A37 (-1.0389, 29.3997) -> (-1.8476, 26.2545) centre (1.0097, 27.1964) ccw projected
  arc A38 (-1.8476, 26.2545) -> (-3.0242, 26.1451) centre (0, 0) ccw projected
  arc A39 (-3.0242, 26.1451) -> (-4.508, 29.1149) centre (-6.2437, 26.3921) ccw projected
  line L12 (-4.508, 29.1149) -> (-4.9482, 28.9989) projected
  arc A40 (-4.9482, 28.9989) -> (-5.3305, 25.774) centre (-2.6243, 27.0883) ccw projected
  arc A41 (-5.3305, 25.774) -> (-6.482, 25.5087) centre (0, 0) ccw projected
  arc A42 (-6.482, 25.5087) -> (-8.3484, 28.2543) centre (-9.7057, 25.3244) ccw projected
  line L13 (-8.3484, 28.2543) -> (-8.7692, 28.0807) projected
  arc A43 (-8.7692, 28.0807) -> (-8.7183, 24.8335) centre (-6.2114, 26.4968) ccw projected
  arc A44 (-8.7183, 24.8335) -> (-9.8241, 24.4172) centre (0, 0) ccw projected
  arc A45 (-9.8241, 24.4172) -> (-12.0399, 26.8894) centre (-12.9945, 23.8048) ccw projected
  line L14 (-12.0399, 26.8894) -> (-12.4338, 26.6613) projected
  arc A46 (-12.4338, 26.6613) -> (-11.9505, 23.4499) centre (-9.6876, 25.4325) ccw projected
  arc A47 (-11.9505, 23.4499) -> (-12.991, 22.8899) centre (0, 0) ccw projected
  arc A48 (-12.991, 22.8899) -> (-15.5165, 25.0448) centre (-16.0514, 21.8604) ccw projected
  line L15 (-15.5165, 25.0448) -> (-15.8764, 24.7661) projected
  arc A49 (-15.8764, 24.7661) -> (-14.9694, 21.6478) centre (-12.991, 23.9143) ccw projected
  arc A50 (-14.9694, 21.6478) -> (-15.926, 20.9541) centre (0, 0) ccw projected
  arc A51 (-15.926, 20.9541) -> (-18.7161, 22.7532) centre (-18.8219, 19.5259) ccw projected
  line L16 (-18.7161, 22.7532) -> (-19.0358, 22.429) projected
  arc A52 (-19.0358, 22.429) -> (-17.7212, 19.4595) centre (-16.0626, 21.9694) ccw projected
  arc A53 (-17.7212, 19.4595) -> (-18.5768, 18.6444) centre (0, 0) ccw projected
  arc A54 (-18.5768, 18.6444) -> (-21.5819, 20.0555) centre (-21.2565, 16.843) ccw projected
  line L17 (-21.5819, 20.0555) -> (-21.8554, 19.6917) projected
  arc A55 (-21.8554, 19.6917) -> (-20.1568, 16.9238) centre (-18.8475, 19.6325) ccw projected
  arc A56 (-20.1568, 16.9238) -> (-20.8961, 16.002) centre (0, 0) ccw projected
  arc A57 (-20.8961, 16.002) -> (-24.0624, 17) centre (-23.3118, 13.8595) ccw projected
  line L18 (-24.0624, 17) -> (-24.2851, 16.603) projected
  arc A58 (-24.2851, 16.603) -> (-22.2327, 14.0862) centre (-21.2961, 16.9452) ccw projected
  arc A59 (-22.2327, 14.0862) -> (-22.8425, 13.0741) centre (0, 0) ccw projected
  arc A60 (-22.8425, 13.0741) -> (-26.1136, 13.6411) centre (-24.9511, 10.6287) ccw projected
  line L19 (-26.1136, 13.6411) -> (-26.2813, 13.2179) projected
  arc A61 (-26.2813, 13.2179) -> (-23.9118, 10.9972) centre (-23.3646, 13.9555) ccw projected
  arc A62 (-23.9118, 10.9972) -> (-24.3813, 9.9128) centre (0, 0) ccw projected
  arc A63 (-24.3813, 9.9128) -> (-27.6988, 10.0388) centre (-26.1452, 7.2082) ccw projected
  line L20 (-27.6988, 10.0388) -> (-27.8086, 9.597) projected
  arc A64 (-27.8086, 9.597) -> (-25.1642, 7.7119) centre (-25.0163, 10.7168) ccw projected
  arc A65 (-25.1642, 7.7119) -> (-25.485, 6.5747) centre (0, 0) ccw projected
  arc A66 (-25.485, 6.5747) -> (-28.7897, 6.2573) centre (-26.8726, 3.6591) ccw projected
  line L21 (-28.7897, 6.2573) -> (-28.8397, 5.8049) projected
  arc A67 (-28.8397, 5.8049) -> (-25.9676, 4.289) centre (-26.2215, 7.2868) ccw projected
  arc A68 (-25.9676, 4.289) -> (-26.1339, 3.1192) centre (0, 0) ccw projected
  arc A69 (-26.1339, 3.1192) -> (-29.3668, 2.3642) centre (-27.1206, 0.0446) ccw projected
  line L22 (-29.3668, 2.3642) -> (-29.356, 1.9091) projected
  arc A70 (-29.356, 1.9091) -> (-26.3076, 0.7896) centre (-26.9587, 3.7268) ccw projected
  arc A71 (-26.3076, 0.7896) -> (-26.3165, -0.392) centre (0, 0) ccw projected
  arc A72 (-26.3165, -0.392) -> (-29.4199, -1.5711) centre (-26.8845, -3.5706) ccw projected
  line L23 (-29.4199, -1.5711) -> (-29.3486, -2.0207) projected
  arc A73 (-29.3486, -2.0207) -> (-26.1781, -2.7239) centre (-27.2149, 0.1003) ccw projected
  arc A74 (-26.1781, -2.7239) -> (-26.0295, -3.8961) centre (0, 0) ccw projected
  arc A75 (-26.0295, -3.8961) -> (-28.948, -5.4784) centre (-26.1687, -7.1221) ccw projected
  line L24 (-28.948, -5.4784) -> (-28.8174, -5.9144) projected
  arc A76 (-28.8174, -5.9144) -> (-25.5815, -6.1888) centre (-26.9855, -3.528) ccw projected
  arc A77 (-25.5815, -6.1888) -> (-25.2779, -7.3307) centre (0, 0) ccw projected
  arc A78 (-25.2779, -7.3307) -> (-27.9595, -9.2879) centre (-24.986, -10.5465) ccw projected
  line L25 (-27.9595, -9.2879) -> (-27.7719, -9.7026) projected
  arc A79 (-27.7719, -9.7026) -> (-24.5283, -9.5432) centre (-26.2745, -7.0933) ccw projected
  arc A80 (-24.5283, -9.5432) -> (-24.0753, -10.6346) centre (0, 0) ccw projected
  arc A81 (-24.0753, -10.6346) -> (-26.4721, -12.9317) centre (-23.3573, -13.7827) ccw projected
  line L26 (-26.4721, -12.9317) -> (-26.2309, -13.3177) projected
  arc A82 (-26.2309, -13.3177) -> (-23.0375, -12.7274) centre (-25.0946, -10.5321) ccw projected
  arc A83 (-23.0375, -12.7274) -> (-22.443, -13.7486) centre (0, 0) ccw projected
  arc A84 (-22.443, -13.7486) -> (-24.5123, -16.3447) centre (-21.3119, -16.7729) ccw projected
  line L27 (-24.5123, -16.3447) -> (-24.2218, -16.6951) projected
  arc A85 (-24.2218, -16.6951) -> (-21.1356, -15.6844) centre (-23.4669, -13.7829) ccw projected
  arc A86 (-21.1356, -15.6844) -> (-20.4103, -16.6173) centre (0, 0) ccw projected
  arc A87 (-20.4103, -16.6173) -> (-22.1151, -19.466) centre (-18.8861, -19.4639) ccw projected
  line L28 (-22.1151, -19.466) -> (-21.7804, -19.7746) projected
  arc A88 (-21.7804, -19.7746) -> (-18.8564, -18.3616) centre (-21.4204, -16.7877) ccw projected
  arc A89 (-18.8564, -18.3616) -> (-18.0133, -19.1894) centre (0, 0) ccw projected
  arc A90 (-18.0133, -19.1894) -> (-19.3232, -22.24) centre (-16.1233, -21.8075) ccw projected
  line L29 (-19.3232, -22.24) -> (-18.9504, -22.5012) projected
  arc A91 (-18.9504, -22.5012) -> (-16.2408, -20.711) centre (-18.9917, -19.493) ccw projected
  arc A92 (-16.2408, -20.711) -> (-15.2949, -21.4191) centre (0, 0) ccw projected
  arc A93 (-15.2949, -21.4191) -> (-16.1865, -24.617) centre (-13.0728, -23.7619) ccw projected
  line L30 (-16.1865, -24.617) -> (-15.7822, -24.8263) projected
  arc A94 (-15.7822, -24.8263) -> (-13.3354, -22.6909) centre (-16.2241, -21.8504) ccw projected
  arc A95 (-13.3354, -22.6909) -> (-12.3035, -23.2666) centre (0, 0) ccw projected
  arc A96 (-12.3035, -23.2666) -> (-12.7609, -26.5548) centre (-9.789, -25.2923) ccw projected
  line L31 (-12.7609, -26.5548) -> (-12.3324, -26.7083) projected
  arc A97 (-12.3324, -26.7083) -> (-10.192, -24.2659) centre (-13.167, -23.8179) ccw projected
  arc A98 (-10.192, -24.2659) -> (-9.0926, -24.6989) centre (0, 0) ccw projected
  arc A99 (-9.0926, -24.6989) -> (-9.1076, -28.0188) centre (-6.3305, -26.3714) ccw projected
  line L32 (-9.1076, -28.0188) -> (-8.6625, -28.1138) projected
  arc A100 (-8.6625, -28.1138) -> (-6.8668, -25.4079) centre (-9.8749, -25.3604) ccw projected
  arc A101 (-6.8668, -25.4079) -> (-5.7194, -25.6905) centre (0, 0) ccw projected
  arc A102 (-5.7194, -25.6905) -> (-5.2918, -28.9827) centre (-2.7591, -26.9799) ccw projected
  line L33 (-5.2918, -28.9827) -> (-4.838, -29.0175) projected
  arc A103 (-4.838, -29.0175) -> (-3.4189, -26.0964) centre (-6.4066, -26.4503) ccw projected
  arc A104 (-3.4189, -26.0964) -> (-2.2442, -26.2236) centre (0, 0) ccw projected
  arc A105 (-2.2442, -26.2236) -> (-1.3816, -29.4294) centre (0.8616, -27.1069) ccw projected
  line L34 (-1.3816, -29.4294) -> (-0.9271, -29.4034) projected
  arc A106 (-0.9271, -29.4034) -> (0.0899, -26.3193) centre (-2.8239, -27.0682) ccw projected
  arc A107 (0.0899, -26.3193) -> (1.2711, -26.2887) centre (0, 0) ccw projected
  arc A108 (1.2711, -26.2887) -> (2.5533, -29.351) centre (4.4669, -26.7502) ccw projected
  line L35 (2.5533, -29.351) -> (3.0002, -29.2647) projected
  arc A109 (3.0002, -29.2647) -> (3.5971, -26.0725) centre (0.8091, -27.2031) ccw projected
  arc A110 (3.5971, -26.0725) -> (4.7637, -25.8847) centre (0, 0) ccw projected
  arc A111 (4.7637, -25.8847) -> (6.4426, -28.7488) centre (7.9925, -25.9161) ccw projected
  line L36 (6.4426, -28.7488) -> (6.8741, -28.6037) projected
  arc A112 (6.8741, -28.6037) -> (7.0401, -25.3604) centre (4.4277, -26.8525) ccw projected
  arc A113 (7.0401, -25.3604) -> (8.1713, -25.0188) centre (0, 0) ccw projected
  arc A114 (8.1713, -25.0188) -> (10.217, -27.6336) centre (11.3755, -24.6196) ccw projected
  line L37 (10.217, -27.6336) -> (10.6252, -27.4322) projected
  arc A115 (10.6252, -27.4322) -> (10.3575, -24.1958) centre (7.9673, -26.0228) ccw projected
  arc A116 (10.3575, -24.1958) -> (11.4331, -23.7065) centre (0, 0) ccw projected
  arc A117 (11.4331, -23.7065) -> (13.809, -26.0252) centre (14.5555, -22.8837) ccw projected
  line L38 (13.809, -26.0252) -> (14.1868, -25.7713) projected
  arc A118 (14.1868, -25.7713) -> (13.4901, -22.5993) centre (11.3647, -24.7286) ccw projected
  arc A119 (13.4901, -22.5993) -> (14.4908, -21.9711) centre (0, 0) ccw projected
  arc A120 (14.4908, -21.9711) -> (17.1546, -23.9525) centre (17.4757, -20.7395) ccw projected
  line L39 (17.1546, -23.9525) -> (17.4952, -23.6504) projected
  arc A121 (17.4952, -23.6504) -> (16.3819, -20.5997) centre (14.5593, -22.9932) ccw projected
  arc A122 (16.3819, -20.5997) -> (17.29, -19.8436) centre (0, 0) ccw projected
  arc A123 (17.29, -19.8436) -> (20.1941, -21.4523) centre (20.0841, -18.2252) ccw projected
  line L40 (20.1941, -21.4523) -> (20.4913, -21.1075) projected
  arc A124 (20.4913, -21.1075) -> (18.9814, -18.2324) centre (17.4941, -20.8475) ccw projected
  arc A125 (18.9814, -18.2324) -> (19.7806, -17.362) centre (0, 0) ccw projected
  arc A126 (19.7806, -17.362) -> (22.8732, -18.5692) centre (22.3341, -15.3856) ccw projected
  line L41 (22.8732, -18.5692) -> (23.1219, -18.1879) projected
  arc A127 (23.1219, -18.1879) -> (21.2422, -15.5397) centre (20.1167, -18.3298) ccw projected
  arc A128 (21.2422, -15.5397) -> (21.9183, -14.5706) centre (0, 0) ccw projected
  arc A129 (21.9183, -14.5706) -> (25.1442, -15.3548) centre (24.1855, -12.2715) ccw projected
  line L42 (25.1442, -15.3548) -> (25.3398, -14.9438) projected
  arc A130 (25.3398, -14.9438) -> (23.1239, -12.5698) centre (22.3803, -15.4849) ccw projected
  arc A131 (23.1239, -12.5698) -> (23.6648, -11.5192) centre (0, 0) ccw projected
  arc A132 (23.6648, -11.5192) -> (26.9664, -11.8665) centre (25.6053, -8.9384) ccw projected
  line L43 (26.9664, -11.8665) -> (27.1055, -11.433) projected
  arc A133 (27.1055, -11.433) -> (24.5929, -9.3755) centre (24.2446, -12.3637) ccw projected
  arc A134 (24.5929, -9.3755) -> (24.989, -8.2622) centre (0, 0) ccw projected
  arc A135 (24.989, -8.2622) -> (28.3075, -8.1663) centre (26.5682, -5.4458) ccw projected
  line L44 (28.3075, -8.1663) -> (28.3875, -7.7182) projected
  arc A136 (28.3875, -7.7182) -> (25.6231, -6.0139) centre (25.6762, -9.0219) ccw projected
  arc A137 (25.6231, -6.0139) -> (25.8672, -4.8578) centre (0, 0) ccw projected
  arc A138 (25.8672, -4.8578) -> (29.1433, -4.3204) centre (27.057, -1.856) ccw projected
  line L45 (29.1433, -4.3204) -> (29.163, -3.8656) projected
  arc A139 (29.163, -3.8656) -> (26.1961, -2.545) centre (26.6496, -5.5191) ccw projected
  arc A140 (26.1961, -2.545) -> (26.2839, -1.3667) centre (0, 0) ccw projected
  arc A141 (26.2839, -1.3667) -> (29.4592, -0.3974) centre (27.063, 1.7669) ccw projected
  line L46 (29.4592, -0.3974) -> (29.418, 0.0559) projected
  circle A142 centre (0, 0) radius 7.5
  line L47 (-29.418, 0.0559) -> (-29.4592, -0.3974)
  arc A143 (-29.4592, -0.3974) -> (-26.1624, -1.3339) centre (-27.063, 1.7669) ccw
  arc A144 (-26.1642, 0.9254) -> (-29.418, 0.0559) centre (-27.1475, -1.9179) ccw
  line L48 (-29.163, -3.8656) -> (-29.1433, -4.3204)
  arc A145 (-29.1433, -4.3204) -> (-25.7511, -4.8091) centre (-27.057, -1.856) ccw
  arc A146 (-26.0541, -2.5702) -> (-29.163, -3.8656) centre (-26.6496, -5.5191) ccw
  line L49 (-28.3875, -7.7182) -> (-28.3075, -8.1663)
  arc A147 (-28.3075, -8.1663) -> (-24.8804, -8.1985) centre (-26.5682, -5.4458) ccw
  arc A148 (-25.4791, -6.0199) -> (-28.3875, -7.7182) centre (-25.6762, -9.0219) ccw
  line L50 (-27.1055, -11.433) -> (-26.9664, -11.8665)
  arc A149 (-26.9664, -11.8665) -> (-23.5656, -11.4416) centre (-25.6053, -8.9384) ccw
  arc A150 (-24.4494, -9.3622) -> (-27.1055, -11.433) centre (-24.2446, -12.3637) ccw
  line L51 (-25.3398, -14.9438) -> (-25.1442, -15.3548)
  arc A151 (-25.1442, -15.3548) -> (-21.8304, -14.4805) centre (-24.1855, -12.2715) ccw
  arc A152 (-22.9834, -12.5375) -> (-25.3398, -14.9438) centre (-22.3803, -15.4849) ccw
  line L52 (-23.1219, -18.1879) -> (-22.8732, -18.5692)
  arc A153 (-22.8732, -18.5692) -> (-19.7055, -17.261) centre (-22.3341, -15.3856) ccw
  arc A154 (-21.1072, -15.489) -> (-23.1219, -18.1879) centre (-20.1167, -18.3298) ccw
  line L53 (-20.4913, -21.1075) -> (-20.1941, -21.4523)
  arc A155 (-20.1941, -21.4523) -> (-17.229, -19.7334) centre (-20.0841, -18.2252) ccw
  arc A156 (-18.8544, -18.1641) -> (-20.4913, -21.1075) centre (-17.4941, -20.8475) ccw
  line L54 (-17.4952, -23.6504) -> (-17.1546, -23.9525)
  arc A157 (-17.1546, -23.9525) -> (-14.4451, -21.8538) centre (-17.4757, -20.7395) ccw
  arc A158 (-16.2651, -20.5151) -> (-17.4952, -23.6504) centre (-14.5593, -22.9932) ccw
  line L55 (-14.1868, -25.7713) -> (-13.809, -26.0252)
  arc A159 (-13.809, -26.0252) -> (-11.4034, -23.5841) centre (-14.5555, -22.8837) ccw
  arc A160 (-13.3856, -22.5) -> (-14.1868, -25.7713) centre (-11.3647, -24.7286) ccw
  line L56 (-10.6252, -27.4322) -> (-10.217, -27.6336)
  arc A161 (-10.217, -27.6336) -> (-8.1582, -24.8936) centre (-11.3755, -24.6196) ccw
  arc A162 (-10.2672, -24.0833) -> (-10.6252, -27.4322) centre (-7.9673, -26.0228) ccw
  line L57 (-6.8741, -28.6037) -> (-6.4426, -28.7488)
  arc A163 (-6.4426, -28.7488) -> (-4.7674, -25.7589) centre (-7.9925, -25.9161) ccw
  arc A164 (-6.9656, -25.2369) -> (-6.8741, -28.6037) centre (-4.4277, -26.8525) ccw
  line L58 (-3.0002, -29.2647) -> (-2.5533, -29.351)
  arc A165 (-2.5533, -29.351) -> (-1.2915, -26.1645) centre (-4.4669, -26.7502) ccw
  arc A166 (-3.5397, -25.9402) -> (-3.0002, -29.2647) centre (-0.8091, -27.2031) ccw
  line L59 (0.9271, -29.4034) -> (1.3816, -29.4294)
  arc A167 (1.3816, -29.4294) -> (2.2074, -26.1032) centre (-0.8616, -27.1069) ccw
  arc A168 (-0.0506, -26.1805) -> (0.9271, -29.4034) centre (2.8239, -27.0682) ccw
  line L60 (4.838, -29.0175) -> (5.2918, -28.9827)
  arc A169 (5.2918, -28.9827) -> (5.6669, -25.5761) centre (2.7591, -26.9799) ccw
  arc A170 (3.4393, -25.9537) -> (4.838, -29.0175) centre (6.4066, -26.4503) ccw
  line L61 (8.6625, -28.1138) -> (9.1076, -28.0188)
  arc A171 (9.1076, -28.0188) -> (9.0253, -24.5925) centre (6.3305, -26.3714) ccw
  arc A172 (6.8679, -25.2637) -> (8.6625, -28.1138) centre (9.8749, -25.3604) ccw
  line L62 (12.3324, -26.7083) -> (12.7609, -26.5548)
  arc A173 (12.7609, -26.5548) -> (12.2226, -23.1702) centre (9.789, -25.2923) ccw
  arc A174 (10.174, -24.1229) -> (12.3324, -26.7083) centre (13.167, -23.8179) ccw
  line L63 (15.7822, -24.8263) -> (16.1865, -24.617)
  arc A175 (16.1865, -24.617) -> (15.2018, -21.3343) centre (13.0728, -23.7619) ccw
  arc A176 (13.2985, -22.5516) -> (15.7822, -24.8263) centre (16.2241, -21.8504) ccw
  line L64 (18.9504, -22.5012) -> (19.3232, -22.24)
  arc A177 (19.3232, -22.24) -> (17.9098, -19.1177) centre (16.1233, -21.8075) ccw
  arc A178 (16.1856, -20.5779) -> (18.9504, -22.5012) centre (18.9917, -19.493) ccw
  line L65 (21.7804, -19.7746) -> (22.1151, -19.466)
  arc A179 (22.1151, -19.466) -> (20.2981, -16.56) centre (18.8861, -19.4639) ccw
  arc A180 (18.784, -18.2369) -> (21.7804, -19.7746) centre (21.4204, -16.7877) ccw
  line L66 (24.2218, -16.6951) -> (24.5123, -16.3447)
  arc A181 (24.5123, -16.3447) -> (22.3243, -13.7068) centre (21.3119, -16.7729) ccw
  arc A182 (21.0471, -15.5705) -> (24.2218, -16.6951) centre (23.4669, -13.7829) ccw
  line L67 (26.2309, -13.3177) -> (26.4721, -12.9317)
  arc A183 (26.4721, -12.9317) -> (23.952, -10.609) centre (23.3573, -13.7827) ccw
  arc A184 (22.9347, -12.6263) -> (26.2309, -13.3177) centre (25.0946, -10.5321) ccw
  line L68 (27.7719, -9.7026) -> (27.9595, -9.2879)
  arc A185 (27.9595, -9.2879) -> (25.1523, -7.3218) centre (24.986, -10.5465) ccw
  arc A186 (24.413, -9.4568) -> (27.7719, -9.7026) centre (26.2745, -7.0933) ccw
  line L69 (28.8174, -5.9144) -> (28.948, -5.4784)
  arc A187 (28.948, -5.4784) -> (25.9038, -3.904) centre (26.1687, -7.1221) ccw
  arc A188 (25.4556, -6.1184) -> (28.8174, -5.9144) centre (26.9855, -3.528) ccw
  line L70 (29.3486, -2.0207) -> (29.4199, -1.5711)
  arc A189 (29.4199, -1.5711) -> (26.193, -0.4165) centre (26.8845, -3.5706) ccw
  arc A190 (26.044, -2.671) -> (29.3486, -2.0207) centre (27.2149, 0.1003) ccw
  line L71 (29.356, 1.9091) -> (29.3668, 2.3642)
  arc A191 (29.3668, 2.3642) -> (26.0148, 3.0784) centre (27.1206, 0.0446) ccw
  arc A192 (26.1676, 0.8242) -> (29.356, 1.9091) centre (26.9587, 3.7268) ccw
  line L72 (28.8397, 5.8049) -> (28.7897, 6.2573)
  arc A193 (28.7897, 6.2573) -> (25.3724, 6.5184) centre (26.8726, 3.6591) ccw
  arc A194 (25.8243, 4.3047) -> (28.8397, 5.8049) centre (26.2215, 7.2868) ccw
  line L73 (27.8086, 9.597) -> (27.6988, 10.0388)
  arc A195 (27.6988, 10.0388) -> (24.2772, 9.842) centre (26.1452, 7.2082) ccw
  arc A196 (25.0201, 7.7083) -> (27.8086, 9.597) centre (25.0163, 10.7168) ccw
  line L74 (26.2813, 13.2179) -> (26.1136, 13.6411)
  arc A197 (26.1136, 13.6411) -> (22.7488, 12.99) centre (24.9511, 10.6287) ccw
  arc A198 (23.7695, 10.9744) -> (26.2813, 13.2179) centre (23.3646, 13.9555) ccw
  line L75 (24.2851, 16.603) -> (24.0624, 17)
  arc A199 (24.0624, 17) -> (20.8144, 15.9062) centre (23.3118, 13.8595) ccw
  arc A200 (22.0946, 14.0446) -> (24.2851, 16.603) centre (21.2961, 16.9452) ccw
  line L76 (21.8554, 19.6917) -> (21.5819, 20.0555)
  arc A201 (21.5819, 20.0555) -> (18.5086, 18.5386) centre (21.2565, 16.843) ccw
  arc A202 (20.0255, 16.8642) -> (21.8554, 19.6917) centre (18.8475, 19.6325) ccw
  line L77 (19.0358, 22.429) -> (18.7161, 22.7532)
  arc A203 (18.7161, 22.7532) -> (15.8725, 20.8402) centre (18.8219, 19.5259) ccw
  arc A204 (17.5991, 19.3829) -> (19.0358, 22.429) centre (16.0626, 21.9694) ccw
  line L78 (15.8764, 24.7661) -> (15.5165, 25.0448)
  arc A205 (15.5165, 25.0448) -> (12.9532, 22.7698) centre (16.0514, 21.8604) ccw
  arc A206 (14.8586, 21.5557) -> (15.8764, 24.7661) centre (12.991, 23.9143) ccw
  line L79 (12.4338, 26.6613) -> (12.0399, 26.8894)
  arc A207 (12.0399, 26.8894) -> (9.8027, 24.2931) centre (12.9945, 23.8048) ccw
  arc A208 (11.8529, 23.3438) -> (12.4338, 26.6613) centre (9.6876, 25.4325) ccw
  line L80 (8.7692, 28.0807) -> (8.3484, 28.2543)
  arc A209 (8.3484, 28.2543) -> (6.4773, 25.3829) centre (9.7057, 25.3244) ccw
  arc A210 (8.6357, 24.7153) -> (8.7692, 28.0807) centre (6.2114, 26.4968) ccw
  line L81 (4.9482, 28.9989) -> (4.508, 29.1149)
  arc A211 (4.508, 29.1149) -> (3.0362, 26.0198) centre (6.2437, 26.3921) ccw
  arc A212 (5.2644, 25.6458) -> (4.9482, 28.9989) centre (2.6243, 27.0883) ccw
  line L82 (1.0389, 29.3997) -> (0.5872, 29.456)
  arc A213 (0.5872, 29.456) -> (-0.4589, 26.1923) centre (2.6702, 26.9888) ccw
  arc A214 (1.7992, 26.1187) -> (1.0389, 29.3997) centre (-1.0097, 27.1964) ccw
  line L83 (-2.889, 29.2759) -> (-3.3442, 29.2714)
  arc A215 (-3.3442, 29.2714) -> (-3.9459, 25.8975) centre (-0.9508, 27.1039) ccw
  arc A216 (-1.6981, 26.1255) -> (-2.889, 29.2759) centre (-4.6256, 26.8191) ccw
  line L84 (-6.7653, 28.6296) -> (-7.2159, 28.5645)
  arc A217 (-7.2159, 28.5645) -> (-7.3625, 25.1404) centre (-4.555, 26.7354) ccw
  arc A218 (-5.1652, 25.666) -> (-6.7653, 28.6296) centre (-8.1589, 25.9633) ccw
  line L85 (-10.5209, 27.4724) -> (-10.9587, 27.3479)